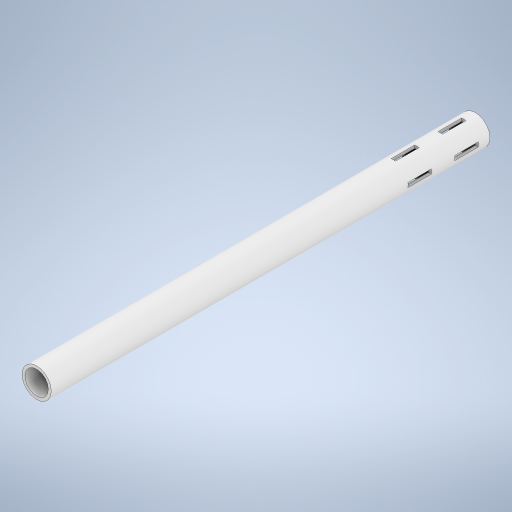
# Autodesk Inventor part: tail
Saved by Autodesk Inventor 2023 (Build 270158000, 158)
## iProperties
Created: 2023-06-06
Part Number: tail
Material: PVC-Piping
Document SubType Name: Modeling
Designer: Ronan
Density: 1.4 g/cm^3
Appearance: Smooth - White
Author: Ronan
Autodesk Inventor part; units mm, degrees
ref_plane "YZ Plane" through (0, 0, 0) normal (1, 0, 0) x (0, 1, 0)
ref_plane "XZ Plane" through (0, 0, 0) normal (0, 1, 0) x (-1, 0, 0)
ref_plane "XY Plane" through (0, 0, 0) normal (0, 0, 1) x (1, 0, 0)
sketch "Sketch1" plane through (0, 0, 0) normal (0, 0, 1) x (1, 0, 0)
  circle A0 centre (0, 0) radius 10
  circle A1 centre (0, 0) radius 8
  dimension "d0" = 16
  dimension "d1" = 20
  constraints: 2 centre point, 2 coincident
  measures "d0" diameter of A1
  measures "d1" diameter of A0
extrude "Extrusion1" add sketch "Sketch1" along normal blind 300
sketch "Sketch2" plane through (0, 0, 0) normal (0, 1, 0) x (-1, 0, 0)
  line L0 (1.5, 8) -> (-1.5, 8)
  line L1 (-1.5, 8) -> (-1.5, 24)
  line L2 (-1.5, 24) -> (1.5, 24)
  line L3 (1.5, 24) -> (1.5, 8)
  line L4 (-1.5, 46.9938) -> (-10, 46.9938)
  line L5 (-10, 0) -> (-10, 300) projected
  line L6 (1.5, 47.6647) -> (10, 47.6647)
  line L7 (10, 0) -> (10, 300) projected
  line L8 (10, 0) -> (-10, 0) projected
  line L9 (1.5, 40) -> (-1.5, 40)
  line L10 (-1.5, 40) -> (-1.5, 56)
  line L11 (-1.5, 56) -> (1.5, 56)
  line L12 (1.5, 56) -> (1.5, 40)
  point P0 (0, 0)
  dimension "d4" = 3
  dimension "d5" = 16
  dimension "d6" = 8
  dimension "d7" = 16
  dimension "d8" = 3
  dimension "d9" = 16
  constraints: 20 end point, 4 horizontal, 4 parallel, 4 point on line, 2 collinear, 2 equal length, 2 perpendicular
  measures "d4" distance between parallel lines of L3 L1
  measures "d5" distance of L2.end L0.start
  measures "d6" distance between parallel lines of L8 L0
  measures "d7" distance between parallel lines of L2 L9
  measures "d8" distance of L9.start L9.end
  measures "d9" distance of L9.end L10.end
extrude "Extrusion2" cut sketch "Sketch2" along normal through all both and the other way through all contours L0 L1 L2 L3 | L10 L11 L12 L9
sketch "Sketch3" plane through (0, 0, 0) normal (1, 0, 0) x (0, 1, 0)
  line L0 (1.5, 8) -> (-1.5, 8)
  line L1 (-1.5, 8) -> (-1.5, 24)
  line L2 (-1.5, 24) -> (1.5, 24)
  line L3 (1.5, 24) -> (1.5, 8)
  line L4 (-1.5, 46.9938) -> (-10, 46.9938)
  line L5 (1.5, 47.6647) -> (10, 47.6647)
  line L6 (10, 0) -> (-10, 0)
  line L7 (1.5, 40) -> (-1.5, 40)
  line L8 (-1.5, 40) -> (-1.5, 56)
  line L9 (-1.5, 56) -> (1.5, 56)
  line L10 (1.5, 56) -> (1.5, 40)
  line L11 (1.5, 18.1726) -> (10, 18.1726)
  line L12 (10, 0) -> (10, 300) projected
  line L13 (-1.5, 20.0085) -> (-10, 20.0085)
  line L14 (-10, 0) -> (-10, 300) projected
  point P0 (0, 0)
  point P1 (0, 0)
  dimension "d12" = 3
  dimension "d13" = 16
  dimension "d15" = 16
  dimension "d16" = 3
  dimension "d17" = 16
  dimension "d18" = 8
  constraints: 26 end point, 6 horizontal, 6 point on line, 4 parallel, 2 collinear, 2 equal length, 2 perpendicular
  measures "d12" distance between parallel lines of L3 L1
  measures "d13" distance of L2.end L0.start
  measures "d15" distance between parallel lines of L2 L7
  measures "d16" distance of L7.start L7.end
  measures "d17" distance of L7.end L8.end
  measures "d18" distance between parallel lines of L6 L0
extrude "Extrusion3" cut sketch "Sketch3" along normal through all both and the other way through all contours L0 L1 L2 L3 | L10 L7 L8 L9
equation "\"BendRadius\" = Thickness"
equation "\"BendReliefWidth\" = Thickness"
equation "\"BendReliefDepth\" = 0.5 * Thickness"
equation "\"CornerReliefSize\" = 4 * Thickness"
equation "\"MinimumRemnant\" = 2 * Thickness"
equation "\"TransitionRadius\" = BendRadius"
equation "\"JacobiRadiusSize\" = BendRadius"
equation "\"GapSize\" = Thickness"
equation "\"Thickness\" = 0.5"
body "Solid1"
